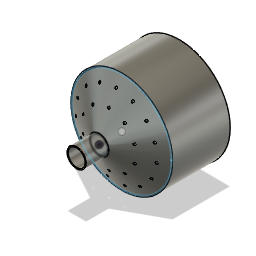
Perlator v2 (Autodesk Fusion 360 design; units mm, degrees)
Autodesk Fusion 360 part; units mm, degrees
sketch "Skizze1" plane through (0, 0, 0) normal (0, 0, 1) x (1, 0, 0)
  circle A0 centre (0, 0) radius 22.5
  dimension "d1" = 45
  constraint coincident A0.centre origin
  measures "d1" diameter of A0
extrude "Extrusion1" add sketch "Skizze1" along normal blind 0.5
sketch "Skizze2" plane through (0, 0, 0.5) normal (0, 0, 1) x (1, 0, 0)
  circle A0 centre (0, 0) radius 22.5
  circle A1 centre (0, 0) radius 22
  dimension "d4" = -0.5
extrude "Extrusion2" add sketch "Skizze2" along normal blind 25
ref_plane "Arbeitsebene1" through (0, 0, 35.5) normal (0, 0, 1) x (1, 0, 0)
sketch "Skizze3" plane through (0, 0, 35.5) normal (0, 0, 1) x (1, 0, 0)
  circle A0 centre (0, 0) radius 4.25
  circle A1 centre (0, 0) radius 3.75
  dimension "d8" = 8.5
  dimension "d9" = -0.5
  constraint coincident A0.centre A1.centre
  measures "d8" diameter of A0
sketch "Skizze4" plane through (0, 0, 25.5) normal (0, 0, 1) x (1, 0, 0)
  circle A0 centre (0, 0) radius 22
  circle A1 centre (0, 0) radius 22.5
  circle A2 centre (0, 0) radius 22
  constraint concentric A0 A2
loft "Erhebung1" add profiles "Skizze4", "Skizze3" section 1 contours A0 A2 | A1 section 2 contours A0 | A1
loft "Erhebung2" cut profiles "Skizze3", "Skizze4" section 1 contours A1 section 2 contours A0 A2
extrude "Extrusion3" add sketch "Skizze3" along normal blind 10
sketch "Skizze5" plane through (0, 0, 0) normal (0, 0, -1) x (-1, 0, 0)
  circle A0 centre (0, 0) radius 22.5
  point P0 (0, 18)
  point P1 (-7.3213, 16.4438)
  point P2 (-13.3766, 12.0444)
  point P3 (-17.119, 5.5623)
  point P4 (-17.9014, -1.8815)
  point P5 (-15.5885, -9)
  point P6 (-10.5801, -14.5623)
  point P7 (-3.7424, -17.6067)
  point P8 (3.7424, -17.6067)
  point P9 (10.5801, -14.5623)
  point P10 (15.5885, -9)
  point P11 (17.9014, -1.8815)
  point P12 (17.119, 5.5623)
  point P13 (13.3766, 12.0444)
  point P14 (7.3213, 16.4438)
  point P15 (0, 12)
  point P16 (-7.0534, 9.7082)
  point P17 (-11.4127, 3.7082)
  point P18 (-11.4127, -3.7082)
  point P19 (-7.0534, -9.7082)
  point P20 (0, -12)
  point P21 (7.0534, -9.7082)
  point P22 (11.4127, -3.7082)
  point P23 (11.4127, 3.7082)
  point P24 (7.0534, 9.7082)
  dimension "d12" = 18
  dimension "d14" = 360
  dimension "d15" = 12
  dimension "d17" = 360
  measures "d12" distance of A0.centre P0
  measures "d15" distance of A0.centre P15
hole "Bohrung1" at (7.0534, 9.7082, 0) at (13.3766, 12.0444, 0) at (17.119, 5.5623, 0) at (0, -12, 0) at (7.0534, -9.7082, 0) at (-7.0534, -9.7082, 0) at (11.4127, 3.7082, 0) at (-10.5801, -14.5623, 0) at (0, 0, 0) at (11.4127, -3.7082, 0) at (17.9014, -1.8815, 0) at (-11.4127, -3.7082, 0) at (-3.7424, -17.6067, 0) at (3.7424, -17.6067, 0) at (15.5885, -9, 0) at (-11.4127, 3.7082, 0) at (0, 0, 0) at (10.5801, -14.5623, 0) at (0, 18, 0) at (-17.119, 5.5623, 0) at (-7.0534, 9.7082, 0) at (-13.3766, 12.0444, 0) at (-7.3213, 16.4438, 0) at (0, 12, 0) at (-17.9014, -1.8815, 0) at (-15.5885, -9, 0) at (7.3213, 16.4438, 0) direction (0, 0, 1) diameter 1 end through all
extrude "Extrusion4" add sketch "Skizze1" along normal blind 0.5
